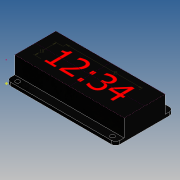
# Autodesk Inventor part: C001
Saved by Autodesk Inventor 2017 (Build 210142000, 142)
## iProperties
Created: 2018-10-19
Part Number: C001
Material: Générique
Document SubType Name: Modeling
Designer: Gilles Mottiez
Density: 1 g/cm^3
Appearance: Anodisé - Noir
Description: Affichage 4 x 7 segments
Author: Gilles Mottiez
Autodesk Inventor part; units mm, degrees
ref_plane "YZ Plane" through (0, 0, 0) normal (1, 0, 0) x (0, 1, 0)
ref_plane "XZ Plane" through (0, 0, 0) normal (0, 1, 0) x (-1, 0, 0)
ref_plane "XY Plane" through (0, 0, 0) normal (0, 0, 1) x (1, 0, 0)
sketch "Sketch1" plane through (0, 0, 0) normal (0, 0, 1) x (1, 0, 0)
  line L0 (0, 0) -> (50.5, 0)
  line L1 (50.5, 0) -> (50.5, 26.8)
  line L2 (50.5, 26.8) -> (0, 26.8)
  line L3 (0, 26.8) -> (0, 0)
  dimension "d0" = 50.5
  dimension "d1" = 26.8
  constraints: 8 end point, 2 parallel, 1 horizontal, 1 perpendicular
  measures "d0" distance of L2.end L1.end
  measures "d1" distance of L1.end L0.end
extrude "Extrusion1" add sketch "Sketch1" along normal blind 1.6
sketch "Esquisse2" plane through (0, 0, 1.6) normal (0, 0, 1) x (1, 0, 0)
  line L0 (0, 0) -> (50.5, 0) construction
  line L1 (50.5, 0) -> (50.5, 26.8) construction
  line L2 (50.5, 26.8) -> (0, 26.8) construction
  line L3 (0, 26.8) -> (0, 0) construction
  line L4 (3.35, 24.9) -> (47.15, 24.9) construction
  line L5 (47.15, 24.9) -> (47.15, 1.9) construction
  line L6 (47.15, 1.9) -> (3.35, 1.9) construction
  line L7 (3.35, 1.9) -> (3.35, 24.9) construction
  line L8 (25.25, 26.8) -> (25.25, 0) construction
  line L9 (0, 13.4) -> (50.5, 13.4) construction
  dimension "d4" = 43.8
  dimension "d5" = 23
  constraints: 12 end point, 4 coincident, 4 midpoint, 2 parallel, 1 horizontal, 1 perpendicular, 2 other
  measures "d4" distance of L4.start L4.end
  measures "d5" distance between parallel lines of L6 L4
hole "Perçage1" at (3.35, 24.9, 1.6) at (3.35, 1.9, 1.6) at (47.15, 24.9, 1.6) at (47.15, 1.9, 1.6) direction (0, 0, -1) diameter 2 end through all
fillet "Congé1" radius 2 4 edges at (0, 26.8, 0.8) (50.5, 26.8, 0.8) (50.5, 0, 0.8) (0, 0, 0.8)
sketch "Esquisse3" plane through (0, 0, 1.6) normal (0, 0, 1) x (1, 0, 0)
  arc A0 (0, 2) -> (2, 0) centre (2, 2) ccw construction
  line L0 (2, 0) -> (48.5, 0) construction
  arc A1 (48.5, 0) -> (50.5, 2) centre (48.5, 2) ccw construction
  line L1 (50.5, 2) -> (50.5, 24.8) construction
  arc A2 (50.5, 24.8) -> (48.5, 26.8) centre (48.5, 24.8) ccw construction
  line L2 (48.5, 26.8) -> (2, 26.8) construction
  arc A3 (2, 26.8) -> (0, 24.8) centre (2, 24.8) ccw construction
  line L3 (0, 24.8) -> (0, 2) construction
  circle A4 centre (47.15, 24.9) radius 1 construction
  circle A5 centre (3.35, 24.9) radius 1 construction
  circle A6 centre (3.35, 1.9) radius 1 construction
  circle A7 centre (47.15, 1.9) radius 1 construction
  line L4 (0, 22.9) -> (50.5, 22.9)
  line L5 (50.5, 22.9) -> (50.5, 3.9)
  line L6 (50.5, 3.9) -> (0, 3.9)
  line L7 (0, 3.9) -> (0, 22.9)
  line L8 (25.25, 26.8) -> (25.25, 0) construction
  line L9 (0, 13.4) -> (50.5, 13.4) construction
  point P0 (0, 0)
  dimension "d14" = 19
  constraints: 12 end point, 4 midpoint, 2 parallel, 2 point on line, 1 horizontal, 1 perpendicular, 1 other
  measures "d14" distance between parallel lines of L6 L4
extrude "Extrusion2" add sketch "Esquisse3" along normal blind 8
sketch "Esquisse4" plane through (0, 0, 0) normal (0, 0, -1) x (-1, 0, 0)
  circle A0 centre (-47.15, 24.9) radius 1 construction
  circle A1 centre (-3.35, 24.9) radius 1 construction
  circle A2 centre (-3.35, 1.9) radius 1 construction
  circle A3 centre (-47.15, 1.9) radius 1 construction
  arc A4 (-2, 0) -> (0, 2) centre (-2, 2) ccw construction
  line L0 (0, 24.8) -> (0, 2) construction
  arc A5 (0, 24.8) -> (-2, 26.8) centre (-2, 24.8) ccw construction
  line L1 (-48.5, 26.8) -> (-2, 26.8) construction
  arc A6 (-48.5, 26.8) -> (-50.5, 24.8) centre (-48.5, 24.8) ccw construction
  line L2 (-50.5, 2) -> (-50.5, 24.8) construction
  arc A7 (-50.5, 2) -> (-48.5, 0) centre (-48.5, 2) ccw construction
  line L3 (-2, 0) -> (-48.5, 0) construction
  line L4 (-34, 17.9) -> (-16, 17.9)
  line L5 (-16, 17.9) -> (-16, 8.9)
  line L6 (-16, 8.9) -> (-34, 8.9)
  line L7 (-34, 8.9) -> (-34, 17.9)
  line L8 (-50.5, 13.4) -> (0, 13.4) construction
  point P0 (0, 0)
  dimension "d17" = 18
  dimension "d18" = 9
  dimension "d19" = 16
  constraints: 10 end point, 2 midpoint, 2 parallel, 1 horizontal, 1 perpendicular, 1 other
  measures "d17" distance of L4.start L4.end
  measures "d18" distance of L4.end L5.end
  measures "d19" distance between parallel lines of L0 L5
extrude "Extrusion3" add sketch "Esquisse4" along normal blind 2.8
sketch "Esquisse5" plane through (0, 0, 0) normal (0, 0, -1) x (-1, 0, 0)
  line L0 (-16, 17.9) -> (-16, 8.9) construction
  line L1 (-16, 8.9) -> (-34, 8.9) construction
  line L2 (-34, 8.9) -> (-34, 17.9) construction
  line L3 (-34, 17.9) -> (-16, 17.9) construction
  circle A0 centre (-47.15, 24.9) radius 1 construction
  circle A1 centre (-3.35, 24.9) radius 1 construction
  circle A2 centre (-3.35, 1.9) radius 1 construction
  circle A3 centre (-47.15, 1.9) radius 1 construction
  arc A4 (-2, 0) -> (0, 2) centre (-2, 2) ccw construction
  line L4 (0, 24.8) -> (0, 2) construction
  arc A5 (0, 24.8) -> (-2, 26.8) centre (-2, 24.8) ccw construction
  line L5 (-48.5, 26.8) -> (-2, 26.8) construction
  arc A6 (-48.5, 26.8) -> (-50.5, 24.8) centre (-48.5, 24.8) ccw construction
  line L6 (-50.5, 2) -> (-50.5, 24.8) construction
  arc A7 (-50.5, 2) -> (-48.5, 0) centre (-48.5, 2) ccw construction
  line L7 (-2, 0) -> (-48.5, 0) construction
  line L8 (-44, 21.9) -> (-16, 21.9)
  line L9 (-16, 21.9) -> (-16, 4.9)
  line L10 (-16, 4.9) -> (-44, 4.9)
  line L11 (-44, 4.9) -> (-44, 21.9)
  line L12 (-16, 17.9) -> (-34, 17.9) construction
  line L13 (-34, 17.9) -> (-34, 8.9) construction
  line L14 (-34, 8.9) -> (-16, 8.9) construction
  line L15 (-16, 8.9) -> (-16, 17.9) construction
  line L16 (-50.5, 13.4) -> (0, 13.4) construction
  point P0 (0, 0)
  dimension "d22" = 28
  dimension "d23" = 17
  constraints: 10 end point, 2 midpoint, 2 parallel, 1 horizontal, 1 perpendicular, 1 vertical alignment, 1 other
  measures "d22" distance of L8.start L8.end
  measures "d23" distance of L10.end L8.start
extrude "Extrusion4" add sketch "Esquisse5" along normal blind 1
sketch "Esquisse6" plane through (0, 0, 1.6) normal (0, 0, 1) x (1, 0, 0)
  line L0 (0, 22.9) -> (50.5, 22.9) construction
  line L1 (50.5, 22.9) -> (50.5, 24.8) construction
  arc A0 (50.5, 24.8) -> (48.5, 26.8) centre (48.5, 24.8) ccw construction
  line L2 (48.5, 26.8) -> (2, 26.8) construction
  arc A1 (2, 26.8) -> (0, 24.8) centre (2, 24.8) ccw construction
  line L3 (0, 24.8) -> (0, 22.9) construction
  circle A2 centre (47.15, 24.9) radius 1 construction
  circle A3 centre (3.35, 24.9) radius 1 construction
  line L4 (21.25, 25) -> (29.25, 25) construction
  line L5 (50.5, 3.9) -> (0, 3.9) construction
  line L6 (0, 3.9) -> (0, 2) construction
  arc A4 (0, 2) -> (2, 0) centre (2, 2) ccw construction
  line L7 (2, 0) -> (48.5, 0) construction
  arc A5 (48.5, 0) -> (50.5, 2) centre (48.5, 2) ccw construction
  line L8 (50.5, 2) -> (50.5, 3.9) construction
  circle A6 centre (3.35, 1.9) radius 1 construction
  circle A7 centre (47.15, 1.9) radius 1 construction
  line L9 (25.25, 26.8) -> (25.25, 0) construction
  point P0 (0, 0)
  point P1 (26.5, 25)
  point P2 (24, 25)
  dimension "d26" = 8
  dimension "d27" = 1.8
  dimension "d28" = 2.5
  constraints: 4 end point, 2 coincident, 2 midpoint, 2 point on line, 2 symmetric about line, 1 horizontal
  measures "d26" distance of L4.start L4.end
  measures "d27" distance between parallel lines of L2 L4
  measures "d28" distance of point (26.5, 25) point (24, 25)
hole "Perçage2" at (21.25, 25, 1.6) at (29.25, 25, 1.6) at (26.5, 25, 1.6) at (24, 25, 1.6) direction (0, 0, -1) diameter 0.8 end through all
sketch "Esquisse7" plane through (0, 0, 9.6) normal (0, 0, 1) x (1, 0, 0)
  line L0 (7.75, 18.4) -> (42.75, 18.4) construction
  line L1 (42.75, 18.4) -> (42.75, 8.4) construction
  line L2 (42.75, 8.4) -> (7.75, 8.4) construction
  line L3 (7.75, 8.4) -> (7.75, 18.4) construction
  line L4 (50.5, 22.9) -> (0, 22.9) construction
  line L5 (0, 22.9) -> (0, 3.9) construction
  line L6 (0, 3.9) -> (50.5, 3.9) construction
  line L7 (50.5, 3.9) -> (50.5, 22.9) construction
  line L8 (25.25, 22.9) -> (25.25, 3.9) construction
  line L9 (0, 13.4) -> (50.5, 13.4) construction
  point P0 (0, 0)
  dimension "d2" = 1.6
  dimension "d36" = 35
  dimension "d37" = 10
  constraints: 4 end point, 4 midpoint, 4 other
  measures "d36" distance of L0.start L0.end
  measures "d37" distance of L2.end L0.start
